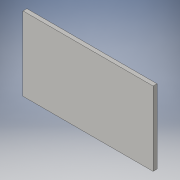
# Autodesk Inventor part: TopWall
Saved by Autodesk Inventor 2016 (Build 200138000, 138)
## iProperties
Created: 2016-05-26
Part Number: TopWall
Material: Generic
Document SubType Name: Modeling
Designer: cutrones
Density: 1 g/cm^3
Appearance: Default
Author: cutrones
Autodesk Inventor part; units mm, degrees
ref_plane "YZ Plane" through (0, 0, 0) normal (1, 0, 0) x (0, 1, 0)
ref_plane "XZ Plane" through (0, 0, 0) normal (0, 1, 0) x (-1, 0, 0)
ref_plane "XY Plane" through (0, 0, 0) normal (0, 0, 1) x (1, 0, 0)
sketch "Sketch1" plane through (0, 0, 0) normal (0, 0, 1) x (1, 0, 0)
  line L0 (0, 0) -> (419.1, 0)
  line L1 (419.1, 0) -> (419.1, 238.125)
  line L2 (419.1, 238.125) -> (0, 238.125)
  line L3 (0, 238.125) -> (0, 0)
  dimension "d0" = 419.1
  dimension "d1" = 238.125
  constraints: 8 end point, 2 parallel, 1 horizontal, 1 perpendicular
  measures "d0" distance of L1.end L2.end
  measures "d1" distance of L0.end L1.end
extrude "Extrusion1" add sketch "Sketch1" along normal mid plane 12.7
equation "\"d0\" = Length"
equation "\"d1\" = Width"
equation "\"d2\" = Thick"
equation "\"Length\" = 419.1"
equation "\"Width\" = 238.125"
equation "\"Thick\" = 12.7"
body "Solid1"
